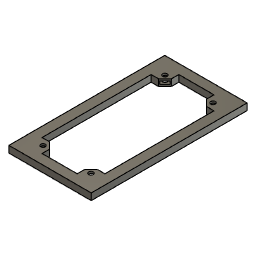
Dimensionen (Autodesk Fusion 360 design; units mm, degrees)
Autodesk Fusion 360 part; units mm, degrees
sketch "Einschubmuttern" plane through (0, 0, 0) normal (0, 1, 0) x (1, 0, 0)
  line L0 (2, 1.1547) -> (0, 2.3094)
  line L1 (0, 2.3094) -> (-2, 1.1547)
  line L2 (-2, 1.1547) -> (-2, -1.1547)
  line L3 (-2, -1.1547) -> (0, -2.3094)
  line L4 (0, -2.3094) -> (2, -1.1547)
  line L5 (2, -1.1547) -> (2, 1.1547)
  line L6 (9.3136, -1.6166) -> (12.1136, -3.2332)
  line L7 (12.1136, -3.2332) -> (14.9136, -1.6166)
  line L8 (14.9136, -1.6166) -> (14.9136, 1.6166)
  line L9 (14.9136, 1.6166) -> (12.1136, 3.2332)
  line L10 (12.1136, 3.2332) -> (9.3136, 1.6166)
  line L11 (9.3136, 1.6166) -> (9.3136, -1.6166)
  circle A0 centre (0, 0) radius 1.15
  circle A1 centre (12.1136, 0) radius 1.65
  circle A2 centre (0, 0) radius 2.25
  circle A3 centre (12.1136, 0) radius 3.25
  line L12 (3.3487, 2.8777) -> (-3.3487, 2.8777)
  line L13 (-3.3487, 2.8777) -> (-3.3487, -2.8777)
  line L14 (-3.3487, -2.8777) -> (3.3487, -2.8777)
  line L15 (3.3487, -2.8777) -> (3.3487, 2.8777)
  line L16 (16.2413, 3.8797) -> (7.986, 3.8797)
  line L17 (7.986, 3.8797) -> (7.986, -3.8797)
  line L18 (7.986, -3.8797) -> (16.2413, -3.8797)
  line L19 (16.2413, -3.8797) -> (16.2413, 3.8797)
  line L20 (-2, 1.1547) -> (-2, 2.8777)
  line L21 (2, 1.1547) -> (2, 2.8777)
  line L22 (9.3136, 1.6166) -> (9.3136, 3.8797)
  line L23 (14.9136, 1.6166) -> (14.9136, 3.8797)
  point P0 (12.1136, 0)
  point P1 (12.1136, 0)
  dimension "d1" = 2
  dimension "d2" = 2.8
  dimension "d3" = 2.3
  dimension "d4" = 3.3
  dimension "d5" = 4.5
  dimension "d6" = 6.5
  constraint coincident A0.centre A2.centre
  constraint coincident P1 P0
  constraint concentric A0 A2
  constraint concentric A1 A3
  constraint horizontal L12
  constraint perpendicular L12 L13
  constraint parallel L12 L14
  constraint parallel L13 L15
  constraint horizontal L16
  constraint perpendicular L16 L17
  constraint parallel L16 L18
  constraint parallel L17 L19
  constraint coincident L12 L20.end
  constraint perpendicular L12 L20
  constraint parallel L5 L21
  constraint coincident L16 L22.end
  constraint perpendicular L16 L22
  constraint coincident L16 L23.end
  constraint perpendicular L16 L23
  measures "d1" distance of A0.centre L5
  measures "d2" distance of P1 L11
  measures "d3" diameter of A0
  measures "d4" diameter of A1
  measures "d5" diameter of A2
  measures "d6" diameter of A3
extrude "Extrude1" add sketch "Einschubmuttern" against normal blind 5 contours L0 L5 A2 | L2 L3 L4 L5 A2 L12 L13 L14 L15 L20 L21 | L0 L1 A2 L12 L20 L21 | L0 L1 L2 L3 L4 L5 A2 | L0 A2 | L5 A2 | L0 L1 A2 | L4 L5 A2 | L1 A2 | L4 A2 | L1 L2 A2 | L3 L4 A2 | L2 A2 | L3 A2 | L2 L3 A2 makes body 1
extrude "Extrude2" cut sketch "Einschubmuttern" against normal blind 1.6 from surface at -2.5 contours L0 L5 A2 | L0 L1 A2 L12 L20 L21 | L0 L1 L2 L3 L4 L5 A2 | L0 A2 | L0 L1 A2 | L4 L5 A2 | L1 A2 | L1 L2 A2 | L3 L4 A2 | L2 L3 A2 bodies 1
extrude "Extrude3" add sketch "Einschubmuttern" against normal blind 6 separate body contours L6 L7 L8 L9 L10 L11 | L6 L7 L8 L11 A3 L22 L23 | L9 L10 A3 L22 L23 | A3 L16 L22 L23 | A3 L16 L17 L18 L19 L22 L23 makes body 2
extrude "Extrude4" cut sketch "Einschubmuttern" against normal blind 2.5 from surface at -3 contours L6 L7 L8 L9 L10 L11 | L9 L10 A3 L22 L23 | A3 L16 L22 L23 bodies 2
chamfer "Chamfer1" distance 1.1 angle 45 1 edges at (-1.0722, 0, -0.4159) on bodies 1
chamfer "Chamfer2" distance 1.6 angle 45 1 edges at (10.5753, 0, -0.5967) on bodies 2
sketch "Sketch2" plane through (0, 0, 0) normal (0, 1, 0) x (1, 0, 0)
  line L0 (2.25, 1.299) -> (0, 2.5981)
  line L1 (0, 2.5981) -> (-2.25, 1.299)
  line L2 (-2.25, 1.299) -> (-2.25, -1.299)
  line L3 (-2.25, -1.299) -> (0, -2.5981)
  line L4 (0, -2.5981) -> (2.25, -1.299)
  line L5 (2.25, -1.299) -> (2.25, 1.299)
  line L6 (14.5056, -1.5877) -> (17.2556, -3.1754)
  line L7 (17.2556, -3.1754) -> (20.0056, -1.5877)
  line L8 (20.0056, -1.5877) -> (20.0056, 1.5877)
  line L9 (20.0056, 1.5877) -> (17.2556, 3.1754)
  line L10 (17.2556, 3.1754) -> (14.5056, 1.5877)
  line L11 (14.5056, 1.5877) -> (14.5056, -1.5877)
  circle A0 centre (0, 0) radius 1.15
  circle A1 centre (17.2556, 0) radius 1.65
  line L12 (5.0227, 4.2637) -> (-5.0227, 4.2637)
  line L13 (-5.0227, 4.2637) -> (-5.0227, -4.2637)
  line L14 (-5.0227, -4.2637) -> (5.0227, -4.2637)
  line L15 (5.0227, -4.2637) -> (5.0227, 4.2637)
  line L16 (11.8758, 5.045) -> (22.6354, 5.045)
  line L17 (22.6354, 5.045) -> (22.6354, -5.045)
  line L18 (22.6354, -5.045) -> (11.8758, -5.045)
  line L19 (11.8758, -5.045) -> (11.8758, 5.045)
  point P0 (17.2556, 0)
  point P1 (17.2556, 0)
  dimension "d19" = 2.25
  dimension "d20" = 2.75
  dimension "d21" = 2.3
  dimension "d22" = 3.3
  constraint coincident A0.centre origin
  constraint coincident P1 P0
  constraint horizontal L12
  constraint perpendicular L12 L13
  constraint parallel L12 L14
  constraint parallel L13 L15
  constraint horizontal L16
  constraint perpendicular L16 L17
  constraint parallel L16 L18
  constraint parallel L17 L19
  measures "d19" distance of A0.centre L5
  measures "d20" distance of P1 L11
  measures "d21" diameter of A0
  measures "d22" diameter of A1
extrude "Extrude5" add sketch "Sketch2" against normal blind 3.5 separate body contours L0 L1 L2 L3 L4 L5 | L6 L7 L8 L9 L10 L11 | L12 L13 L14 L15 | L16 L17 L18 L19 makes body 3 at (3.7318, 0, 0) makes body 4 at (13.1191, 0, 0)
extrude "Extrude6" cut sketch "Sketch2" against normal blind 1.8 contours L0 L1 L2 L3 L4 L5 bodies 3
extrude "Extrude7" cut sketch "Sketch2" against normal blind 2.5 contours L6 L7 L8 L9 L10 L11 bodies 4
sketch "TOF" plane through (0, 0, 0) normal (0, 1, 0) x (1, 0, 0)
  line L0 (5.5969, 3.1885) -> (5.5969, 0.7636)
  line L1 (-8.8031, 0.7636) -> (-6.7031, -0.4488)
  line L2 (8.1469, -1.524) -> (8.1469, -1.6348)
  circle A0 centre (-1.8031, 1.976) radius 2.6
  line L3 (-6.7031, 4.4009) -> (-8.8031, 3.1885)
  line L4 (-9.6031, 2.476) -> (-9.6031, 1.476)
  line L5 (9.7969, 3.1885) -> (7.6969, 4.4009)
  circle A1 centre (7.6969, 1.976) radius 1.15
  arc A2 (-9.6031, 1.476) -> (-7.3062, -1.4404) centre (-6.6031, 1.476) ccw
  line L6 (-15.7687, -9.3798) -> (-15.7687, 8.4065)
  line L7 (0.4969, -1.524) -> (-7.1531, -1.524)
  line L8 (-8.8031, 3.1885) -> (-8.8031, 0.7636)
  line L9 (-7.1531, -1.524) -> (-7.1531, -1.6348)
  line L10 (5.5969, 0.7636) -> (7.6969, -0.4488)
  line L11 (5.3969, -0.624) -> (5.3969, 4.576)
  line L12 (-4.4031, 1.976) -> (-1.8031, 1.976)
  line L13 (0.4969, -6.024) -> (0.4969, -1.524)
  line L14 (-6.7031, -0.4488) -> (-4.6031, 0.7636)
  arc A3 (8.3, -1.4404) -> (8.1469, -1.6348) centre (8.3469, -1.6348) ccw
  circle A4 centre (-6.7031, 1.976) radius 1.15
  circle A5 centre (-6.7031, 1.976) radius 2.3
  line L15 (-4.4031, -0.624) -> (5.3969, -0.624)
  circle A6 centre (2.7969, 1.976) radius 2.6
  line L16 (-15.7687, 8.4065) -> (15.9174, 8.4065)
  line L17 (9.7969, 0.7636) -> (9.7969, 3.1885)
  line L18 (-4.4031, 4.576) -> (-4.4031, -0.624)
  arc A7 (-6.6031, 5.476) -> (-9.6031, 2.476) centre (-6.6031, 2.476) ccw
  arc A8 (10.5969, 2.476) -> (7.5969, 5.476) centre (7.5969, 2.476) ccw
  circle A9 centre (7.6969, 1.976) radius 2.3
  line L19 (-4.6031, 3.1885) -> (-6.7031, 4.4009)
  line L20 (-7.1531, -6.024) -> (0.4969, -6.024)
  line L21 (15.9174, 8.4065) -> (15.9174, -9.3798)
  line L22 (8.1469, -6.024) -> (0.4969, -6.024)
  line L23 (10.5969, 1.476) -> (10.5969, 2.476)
  line L24 (7.6969, -0.4488) -> (9.7969, 0.7636)
  line L25 (-7.1531, -1.524) -> (-7.1531, -6.024)
  line L26 (5.3969, 4.576) -> (-4.4031, 4.576)
  line L27 (5.3969, 1.976) -> (2.7969, 1.976)
  line L28 (-4.6031, 0.7636) -> (-4.6031, 3.1885)
  line L29 (8.1469, -1.524) -> (8.1469, -6.024)
  arc A10 (8.3, -1.4404) -> (10.5969, 1.476) centre (7.5969, 1.476) ccw
  line L30 (7.5969, 5.476) -> (-6.6031, 5.476)
  line L31 (7.6969, 4.4009) -> (5.5969, 3.1885)
  line L32 (-6.7031, 1.976) -> (7.6969, 1.976)
  arc A11 (-7.1531, -1.6348) -> (-7.3062, -1.4404) centre (-7.3531, -1.6348) ccw
  line L33 (15.9174, -9.3798) -> (-15.7687, -9.3798)
  line L34 (-6.6031, -1.524) -> (7.5969, -1.524)
  line L35 (0.4969, -6.024) -> (0.4969, -1.524)
  line L36 (0.4969, -1.524) -> (8.1469, -1.524)
  point P0 (0.4969, 1.976)
  point P1 (0.4969, 1.976)
  point P2 (7.6969, 1.976)
  point P3 (-6.7031, 1.976)
  dimension "d29" = 2.3
  dimension "d30" = 14.4
  dimension "d31" = 2.3
  dimension "d32" = 9.8
  dimension "d33" = 5.2
  dimension "d34" = 2.6
  dimension "d35" = 2.6
  dimension "d38" = 3
  dimension "d39" = 7.65
  dimension "d40" = 4.5
  dimension "d41" = 7.65
  dimension "d42" = 0.2
  dimension "d43" = 0.2
  dimension "d44" = 4.6
  dimension "d45" = 4.6
  dimension "d46" = 2.1
  dimension "d47" = 2.1
  constraint coincident P3 A4.centre
  constraint horizontal L32
  constraint coincident P2 A1.centre
  constraint horizontal L26
  constraint perpendicular L18 L26
  constraint parallel L15 L26
  constraint parallel L11 L18
  constraint midpoint P1 L32
  constraint midpoint L12.start L18
  constraint perpendicular L12 L18
  constraint coincident A0.centre L12.end
  constraint coincident L12.start A0
  constraint midpoint L27.start L11
  constraint perpendicular L11 L27
  constraint coincident A6.centre L27.end
  constraint coincident L27.start A6
  constraint horizontal L30
  constraint perpendicular L4 L30
  constraint parallel L30 L34
  constraint parallel L4 L23
  constraint coincident P1 P0
  constraint tangent A7 L30
  constraint tangent L4 A7
  constraint tangent A2 L34
  constraint tangent L4 A2
  constraint equal A2 A7
  constraint tangent A10 L34
  constraint tangent L23 A10
  constraint equal A7 A10
  constraint tangent A8 L30
  constraint tangent A8 L23
  constraint equal A7 A8
  constraint horizontal L36
  constraint vertical L29
  constraint horizontal L22
  constraint vertical L13
  constraint midpoint L7.start L34
  constraint horizontal L7
  constraint vertical L25
  constraint horizontal L20
  constraint vertical L35
  constraint perpendicular L7 L9
  constraint perpendicular L2 L36
  constraint tangent L2 A3
  constraint tangent A3 A10
  constraint tangent L9 A11
  constraint tangent A2 A11
  constraint horizontal L16
  constraint vertical L21
  constraint horizontal L33
  constraint vertical L6
  constraint coincident A1.centre A9.centre
  measures "d29" diameter of A4
  measures "d30" distance of P3 P2
  measures "d31" diameter of A1
  measures "d32" distance of L15.start L11.start
  measures "d33" distance of L15.start L18.start
  measures "d34" distance of L12.start A0.centre
  measures "d35" distance of A6.centre L27.start
  measures "d38" radius of A7
  measures "d39" distance of L7.start L2.start
  measures "d40" distance of L7.start L13.start
  measures "d41" distance of L7.start L7.end
  measures "d42" radius of A3
  measures "d43" radius of A11
  measures "d44" diameter of A5
  measures "d45" diameter of A9
  measures "d46" distance of P2 L17
  measures "d47" distance of P3 L28
extrude "TOF (1)" add sketch "TOF" against normal blind 1.3 separate body contours L0 A9 L31 | A5 L28 L32 | A5 L28 L32 | L11 L15 A6 | L11 A6 L26 | L0 L5 L10 L17 A9 L24 L31 | L0 A9 L32 | A9 L31 | L0 A9 L32 | L5 A9 L31 | L0 L10 A9 | L5 A9 | L10 A9 | A0 L18 L26 | A0 L15 L18 | L5 L17 A9 | L10 A9 L24 | L17 A9 | A9 L24 | L1 L3 L8 L14 A5 L19 L28 | A5 L19 L28 | L14 A5 L28 | L17 A9 L24 | A5 L19 | L14 A5 | L3 A5 L19 | L1 L14 A5 | L3 A5 | L1 A5 | L3 L8 A5 | L1 L8 A5 | L8 A5 | L2 L4 A2 L7 L9 A3 A7 A8 L23 L25 L29 A10 L30 A11 L34 L36 | L2 L13 L22 L29 L34 L35 L36 | L7 L9 L13 L20 L25 L34 L35 | L6 L16 L21 L33 makes body 5
extrude "TOF (2)" add sketch "TOF" along normal blind 2 contours L6 L16 L21 L33 bodies 5
chamfer "TOF (3)" distance 1.15 angle 45 2 edges at (-7.7753, -1.3, -1.5602) (6.6247, -1.3, -1.5602) on bodies 5
sketch "USB-C Buchse" plane through (0, 0, 0) normal (0, 1, 0) x (1, 0, 0)
  line L0 (0, 0) -> (14.25, 0)
  line L1 (14.25, 0) -> (14.25, -5.7)
  line L2 (14.25, -5.7) -> (0, -5.7)
  line L3 (0, -5.7) -> (0, 0)
  line L4 (20.5801, -12.0301) -> (-6.3301, -12.0301)
  line L5 (-6.3301, -12.0301) -> (-6.3301, 6.3301)
  line L6 (-6.3301, 6.3301) -> (20.5801, 6.3301)
  line L7 (20.5801, 6.3301) -> (20.5801, -12.0301)
  dimension "d53" = 14.25
  dimension "d54" = 5.7
  dimension "d55" = -6.3301
  constraint horizontal L0
  constraint vertical L1
  constraint horizontal L2
  constraint vertical L3
  constraint coincident L0.start L3.end
  measures "d53" distance of L0.start L0.end
  measures "d54" distance of L0.start L2.end
extrude "Extrude10" add sketch "USB-C Buchse" against normal blind 3 separate body makes body 6
sketch "USB-C Stecker" plane through (0, 0, 0) normal (0, 1, 0) x (1, 0, 0)
  line L0 (0, 0) -> (9, 0)
  line L1 (9, 0) -> (9, -3) construction
  line L2 (9, -3) -> (0, -3)
  line L3 (0, -3) -> (0, 0) construction
  line L4 (12, -6) -> (-3, -6)
  line L5 (-3, -6) -> (-3, 3)
  line L6 (-3, 3) -> (12, 3)
  line L7 (12, 3) -> (12, -6)
  line L8 (0, -1.5) -> (1.5, -1.5) construction
  line L9 (9, -1.5) -> (7.5, -1.5) construction
  circle A0 centre (1.5, -1.5) radius 1.5
  circle A1 centre (7.5, -1.5) radius 1.5
  dimension "d58" = 9
  dimension "d59" = 3
  dimension "d60" = -3
  dimension "d61" = 1.5
  dimension "d62" = 1.5
  constraint horizontal L0
  constraint vertical L1
  constraint horizontal L2
  constraint vertical L3
  constraint coincident L0.start L3.end
  constraint midpoint L3 L8.start
  constraint perpendicular L3 L8
  constraint midpoint L1 L9.start
  constraint perpendicular L1 L9
  constraint coincident L8.end A0.centre
  constraint coincident L8.start A0
  constraint coincident L9.end A1.centre
  constraint coincident L9.start A1
  measures "d58" distance of L0.start L0.end
  measures "d59" distance of L0.start L2.end
  measures "d61" distance of L8.start L8.end
  measures "d62" distance of L9.start L9.end
extrude "Extrude11" add sketch "USB-C Stecker" against normal blind 3 separate body makes body 7
sketch "ESP32-C6-DevKit" plane through (0, 0, 0) normal (0, 1, 0) x (1, 0, 0)
  circle A0 centre (24.0333, -6.3894) radius 1.25
  circle A1 centre (24.0333, -27.2477) radius 1.25
  line L0 (28.261, -31.6633) -> (-30.2467, -31.6633)
  line L1 (-29.9467, -3.9685) -> (-29.9467, -29.6686)
  line L2 (28.261, -3.3133) -> (28.261, -31.6633)
  line L3 (30.5691, -27.2494) -> (24.0333, -27.2494) construction
  circle A2 centre (-27.1863, -27.2477) radius 1.25
  line L4 (26.761, -3.9685) -> (-29.9467, -3.9685)
  line L5 (26.761, -29.6686) -> (26.761, -3.9685)
  line L6 (-28.9563, -27.2477) -> (25.1533, -27.2477) construction
  line L7 (28.261, -2.4685) -> (-30.5467, -2.4685)
  line L8 (25.1533, -6.3894) -> (-28.9563, -6.3894) construction
  line L9 (-29.9467, -29.6686) -> (26.761, -29.6686)
  circle A3 centre (-27.1863, -6.3894) radius 1.25
  line L10 (-29.3467, -29.6686) -> (-29.9467, -29.6686)
  line L11 (24.0333, -5.1352) -> (24.0333, -29.4977) construction
  line L12 (-29.6467, -3.9685) -> (-29.9467, -3.9685)
  line L13 (25.1533, -14.9026) -> (25.1533, -6.3894) construction
  line L14 (-27.1863, -5.1352) -> (-27.1863, -29.4977) construction
  line L15 (-28.9563, -6.3894) -> (-28.9563, -27.2477) construction
  line L16 (30.5691, -6.3894) -> (30.5691, -27.2494) construction
  line L17 (24.0333, -27.2494) -> (24.0333, -6.3894) construction
  line L18 (24.0333, -6.3894) -> (30.5691, -6.3894) construction
  line L19 (-27.1863, -25.0177) -> (-27.0488, -25.0177)
  line L20 (28.261, -3.3133) -> (28.261, -2.4685)
  line L21 (-25.1863, -5.2347) -> (-27.1863, -4.08)
  line L22 (-27.1863, -4.08) -> (-29.1863, -5.2347)
  line L23 (-29.1863, -5.2347) -> (-29.1863, -7.5441)
  line L24 (-29.1863, -7.5441) -> (-27.1863, -8.6988)
  line L25 (-27.1863, -8.6988) -> (-25.1863, -7.5441)
  line L26 (-25.1863, -7.5441) -> (-25.1863, -5.2347)
  line L27 (-25.1863, -5.2347) -> (-25.1863, -2.4685)
  line L28 (-29.1863, -5.2347) -> (-29.1863, -2.4685)
  line L29 (26.0333, -5.2347) -> (24.0333, -4.08)
  line L30 (24.0333, -4.08) -> (22.0333, -5.2347)
  line L31 (22.0333, -5.2347) -> (22.0333, -7.5441)
  line L32 (22.0333, -7.5441) -> (24.0333, -8.6988)
  line L33 (24.0333, -8.6988) -> (26.0333, -7.5441)
  line L34 (26.0333, -7.5441) -> (26.0333, -5.2347)
  line L35 (26.0344, -26.0949) -> (24.0354, -24.9383)
  line L36 (24.0354, -24.9383) -> (22.0344, -26.0912)
  line L37 (22.0344, -26.0912) -> (22.0322, -28.4006)
  line L38 (22.0322, -28.4006) -> (24.0312, -29.5571)
  line L39 (24.0312, -29.5571) -> (26.0322, -28.4043)
  line L40 (26.0322, -28.4043) -> (26.0344, -26.0949)
  line L41 (-25.1863, -26.093) -> (-27.1863, -24.9383)
  line L42 (-27.1863, -24.9383) -> (-29.1863, -26.093)
  line L43 (-29.1863, -26.093) -> (-29.1863, -28.4024)
  line L44 (-29.1863, -28.4024) -> (-27.1863, -29.5571)
  line L45 (-27.1863, -29.5571) -> (-25.1863, -28.4024)
  line L46 (-25.1863, -28.4024) -> (-25.1863, -26.093)
  line L47 (-25.1863, -28.4024) -> (-25.1863, -31.6633)
  line L48 (-29.1863, -28.4024) -> (-29.1863, -31.6633)
  line L49 (22.0333, -5.2347) -> (22.0333, -2.4685)
  line L50 (26.0333, -5.2347) -> (26.0333, -2.4685)
  line L51 (26.0322, -28.4043) -> (26.0322, -31.6633)
  line L52 (22.0322, -28.4006) -> (22.0322, -31.6633)
  line L53 (-29.9467, -17.4783) -> (-30.5467, -17.4783)
  line L54 (-30.5467, -21.9783) -> (-29.9467, -21.9783)
  line L55 (-29.9467, -21.9783) -> (-29.9467, -17.4783)
  line L56 (-29.9467, -17.4783) -> (-30.5467, -17.4783)
  line L57 (-30.5467, -12.9783) -> (-29.9467, -12.9783)
  line L58 (-29.9467, -12.9783) -> (-29.9467, -17.4783)
  line L59 (-24.9563, -29.6686) -> (-24.7063, -29.6686)
  line L60 (-24.7063, -29.6686) -> (-24.7063, -4.4633)
  line L61 (21.6533, -3.9685) -> (21.4033, -3.9685)
  line L62 (-24.7063, -4.4633) -> (-24.7063, -3.9685)
  line L63 (21.5526, -3.9685) -> (21.5526, -29.6686)
  line L64 (-30.5467, -2.4685) -> (-30.7467, -2.4685)
  line L65 (-30.7467, -2.4685) -> (-30.7467, -31.6633)
  line L66 (-30.7467, -31.6633) -> (-30.2467, -31.6633)
  line L67 (-30.5467, -12.9783) -> (-30.7467, -12.9783)
  line L68 (-30.5467, -21.9783) -> (-30.7467, -21.9783)
  line L69 (-30.5467, -17.4783) -> (-30.7467, -17.4783)
  point P0 (-28.9563, -17.3164)
  point P1 (-1.5967, -17.8133)
  point P2 (-28.9563, -29.4977)
  point P3 (-27.1863, -6.3894)
  point P4 (24.0333, -6.3894)
  point P5 (24.0333, -27.2477)
  point P6 (-27.1863, -27.2477)
  dimension "d67" = 2.5
  dimension "d68" = 2.5
  dimension "d69" = 2.5
  dimension "d70" = 2.5
  dimension "d137" = 20.86
  dimension "d138" = 2
  dimension "d139" = 2
  dimension "d140" = 2
  dimension "d141" = 2
  dimension "d142" = 4.5
  dimension "d143" = 4.5
  constraint horizontal L8
  constraint perpendicular L8 L15
  constraint parallel L13 L15
  constraint horizontal L6
  constraint vertical L11
  constraint vertical L14
  constraint coincident P3 L14
  constraint coincident P3 L8
  constraint coincident P4 L8
  constraint coincident P4 L11
  constraint coincident P5 L6
  constraint coincident P5 L11
  constraint coincident P6 L6
  constraint coincident P6 L14
  constraint horizontal L4
  constraint parallel L4 L9
  constraint horizontal L12
  constraint vertical L1
  constraint horizontal L10
  constraint coincident L12.start L4
  constraint coincident L10.start L9
  constraint horizontal L0
  constraint vertical L2
  constraint coincident L59.start L9
  constraint coincident L19.start L14
  constraint coincident L61.start L4
  constraint horizontal L18
  constraint vertical L16
  constraint horizontal L3
  constraint vertical L17
  constraint coincident P4 A0.centre
  constraint perpendicular L7 L20
  constraint coincident P3 A3.centre
  constraint coincident L7 L27.end
  constraint perpendicular L7 L27
  constraint coincident L7 L28.end
  constraint perpendicular L7 L28
  constraint coincident P5 A1.centre
  constraint coincident P6 A2.centre
  constraint coincident L0 L47.end
  constraint perpendicular L0 L47
  constraint coincident L0 L48.end
  constraint perpendicular L0 L48
  constraint coincident L7 L49.end
  constraint perpendicular L7 L49
  constraint coincident L7 L50.end
  constraint perpendicular L7 L50
  constraint coincident L0 L51.end
  constraint perpendicular L0 L51
  constraint coincident L0 L52.end
  constraint perpendicular L0 L52
  constraint horizontal L53
  constraint horizontal L54
  constraint vertical L55
  constraint horizontal L56
  constraint horizontal L57
  constraint vertical L58
  constraint horizontal L59
  constraint vertical L60
  constraint horizontal L61
  constraint coincident L41 L19.end
  constraint coincident L4 L62.end
  constraint perpendicular L4 L62
  constraint coincident L4 L63.start
  constraint coincident L9 L63.end
  constraint perpendicular L9 L63
  constraint coincident L1 L53.start
  constraint horizontal L64
  constraint vertical L65
  constraint horizontal L66
  constraint coincident L65 L67.end
  constraint perpendicular L65 L67
  constraint coincident L65 L68.end
  constraint perpendicular L65 L68
  constraint coincident L65 L69.end
  constraint perpendicular L65 L69
  measures "d67" diameter of A3
  measures "d68" diameter of A0
  measures "d69" diameter of A1
  measures "d70" diameter of A2
  measures "d137" distance of L16.start L3.start
  measures "d138" distance of P3 L26
  measures "d139" distance of P4 L34
  measures "d140" distance of P5 L40
  measures "d141" distance of P6 L46
  measures "d142" distance of L53.start L54.end
  measures "d143" distance of L53.start L57.end
extrude "Boden" add sketch "ESP32-C6-DevKit" against normal blind 1 separate body makes body 8
extrude "Ablage" add sketch "ESP32-C6-DevKit" along normal blind 9.3 contours L4 L5 L9 L31 L32 L33 L34 L35 L36 L37 L40 L49 L50 L51 L52 L61 L63 | L9 L38 L39 L51 L52 | L35 L36 L37 L38 L39 L40 | L1 L4 L9 L10 L12 L23 L24 L25 L26 L27 L28 L41 L42 L43 L46 L47 L48 L55 L58 L59 L60 L62 | L9 L44 L45 L47 L48 | L4 L29 L30 L49 L50 | L41 L42 L43 L44 L45 L46 | L29 L30 L31 L32 L33 L34 | L4 L21 L22 L27 L28 | L21 L22 L23 L24 L25 L26 bodies 8
extrude "Extrude15" add sketch "ESP32-C6-DevKit" along normal blind 15.9 contours L0 L2 L4 L5 L7 L9 L20 L50 L51 | L0 L9 L51 L52 | L0 L9 L47 L52 L59 | L0 L9 L47 L48 | L4 L7 L49 L50 | L0 L1 L9 L10 L48 L54 L65 L66 L68 | L4 L7 L27 L49 L61 | L4 L7 L27 L28 | L1 L4 L7 L12 L28 L57 L64 L65 L67 | L1 L53 L54 L55 L56 L65 L68 L69 | L1 L53 L56 L57 L58 L65 L67 L69 bodies 8
extrude "Einschubmutter" cut sketch "ESP32-C6-DevKit" against normal blind 1.6 from surface at 8.3 contours L0 L9 L51 L52 | L9 L38 L39 L51 L52 | L0 L9 L47 L48 | L35 L36 L37 L38 L39 L40 | L4 L7 L49 L50 | L9 L44 L45 L47 L48 | L4 L29 L30 L49 L50 | L41 L42 L43 L44 L45 L46 | L4 L7 L27 L28 | L29 L30 L31 L32 L33 L34 | L4 L21 L22 L27 L28 | L21 L22 L23 L24 L25 L26 bodies 8
sketch "ESP32-DevKit Wand Buchse" plane through (-30.7467, 0, 0) normal (-1, 0, 0) x (0, 0, 1)
  line L0 (2.4685, 15.9) -> (2.4685, -1)
  line L1 (2.4685, -1) -> (31.6633, -1)
  line L2 (31.6633, -1) -> (31.6633, 15.9)
  line L3 (31.6633, 15.9) -> (2.4685, 15.9)
  line L4 (3.9685, 9.3) -> (29.6686, 9.3)
  line L5 (12.3186, 9.3) -> (21.078, 9.3)
  line L6 (21.078, 10.9) -> (12.3186, 10.9)
  line L7 (12.3186, 10.9) -> (12.3186, 9.3)
  line L8 (12.3186, 10.9) -> (21.3186, 10.9)
  line L9 (21.3186, 10.9) -> (21.3186, 13.9)
  line L10 (21.3186, 13.9) -> (12.3186, 13.9)
  line L11 (12.3186, 13.9) -> (12.3186, 10.9)
  line L12 (12.3186, 12.4) -> (13.8186, 12.4)
  circle A0 centre (13.8186, 12.4) radius 1.5
  line L13 (21.3186, 12.4) -> (19.8186, 12.4)
  circle A1 centre (19.8186, 12.4) radius 1.5
  dimension "d271" = 1.6
  dimension "d272" = 3
  dimension "d273" = 1.5
  dimension "d274" = 1.5
  constraint horizontal L5
  constraint horizontal L6
  constraint vertical L7
  constraint coincident L4 L5.start
  constraint horizontal L8
  constraint vertical L9
  constraint horizontal L10
  constraint vertical L11
  constraint midpoint L11 L12.start
  constraint perpendicular L11 L12
  constraint coincident L12.end A0.centre
  constraint coincident L12.start A0
  constraint midpoint L9 L13.start
  constraint perpendicular L9 L13
  constraint coincident L13.end A1.centre
  constraint coincident L13.start A1
  measures "d271" distance of L5.start L6.end
  measures "d272" distance of L6.end L10.end
  measures "d273" distance of L12.start L12.end
  measures "d274" distance of L13.start L13.end
extrude "Extrude27" cut sketch "ESP32-DevKit Wand Buchse" along normal mid plane 6 contours L6 L8 L10 A0 A1 | A1 | A0 bodies 8
sketch "LED-Ring" plane through (0, 0, 0) normal (0, 1, 0) x (1, 0, 0)
  circle A0 centre (0, 0) radius 18
  circle A1 centre (0, 0) radius 20.7 construction
  line L0 (0, 0) -> (0, -20.7) construction
  line L1 (2.8, -17.9) -> (-2.8, -17.9)
  line L2 (-2.8, -17.9) -> (-2.8, -23.5)
  line L3 (-2.8, -23.5) -> (2.8, -23.5)
  line L4 (2.8, -23.5) -> (2.8, -17.9)
  line L5 (2.8, -17.9) -> (-2.8, -23.5) construction
  line L6 (-2.8, -17.9) -> (2.8, -23.5) construction
  circle A2 centre (0, -20.7) radius 1.75
  line L7 (0, 0) -> (22.6032, -22.6032) construction
  line L8 (0, 0) -> (31.9658, 0) construction
  circle A3 centre (0, 0) radius 23.18 construction
  circle A4 centre (16.3907, -16.3907) radius 1.25
  circle A5 centre (0, 0) radius 32.5
  circle A6 centre (16.3907, -16.3907) radius 2.25
  line L9 (7.6403, -23.8039) -> (7.6403, -31.5892)
  line L10 (-7.6403, -31.5892) -> (-7.6403, -23.8039)
  arc A7 (-7.6403, -23.8039) -> (7.6403, -23.8039) centre (0, 0) ccw
  arc A8 (17.6777, -17.6777) -> (16.6799, -18.6221) centre (0, 0) ccw
  line L11 (-2.8, -23.5) -> (2.8, -23.5)
  line L12 (2.8, -23.5) -> (2.8, -25.3)
  line L13 (2.8, -25.3) -> (-2.8, -25.3)
  line L14 (-2.8, -25.3) -> (-2.8, -23.5)
  point P0 (0, -20.7)
  point P1 (0, -25)
  dimension "d170" = 50
  dimension "d171" = 36
  dimension "d172" = 2.7
  dimension "d173" = 5.6
  dimension "d174" = 5.6
  dimension "d175" = 3.5
  dimension "d176" = 45
  dimension "d178" = 2.5
  dimension "d179" = 65
  dimension "d190" = 4.5
  dimension "d267" = 1.8
  constraint coincident A0.centre A1.centre
  constraint concentric A0 A8
  constraint coincident A1 P0
  constraint vertical L0
  constraint horizontal L1
  constraint perpendicular L1 L2
  constraint parallel L1 L3
  constraint parallel L2 L4
  constraint coincident L5 P0
  constraint coincident L6 P0
  constraint coincident P0 L0.end
  constraint horizontal L8
  constraint coincident L7 A4.centre
  constraint coincident A3 A4.centre
  constraint concentric A5 A8
  constraint concentric A4 A6
  constraint parallel L9 L10
  constraint coincident P1 A8
  constraint coincident L9.start A8
  constraint coincident L10.end A8
  constraint coincident A5 L10.start
  constraint coincident A5 L9.end
  constraint coincident A6 A8.end
  constraint concentric A3 A8
  constraint coincident L7 A8.start
  constraint horizontal L11
  constraint vertical L12
  constraint horizontal L13
  constraint vertical L14
  measures "d170" diameter of A8
  measures "d171" diameter of A0
  measures "d173" distance of L2.end L3.end
  measures "d174" distance of L1.end L2.end
  measures "d175" diameter of A2
  measures "d176" angle of L7 L8
  measures "d178" diameter of A4
  measures "d179" diameter of A5
  measures "d190" diameter of A6
  measures "d267" distance of L2.end L13.end
extrude "LED-Ring Base Plate" add sketch "LED-Ring" against normal blind 2 separate body contours A0 L1 | A0 L1 L2 L4 A6 A7 A8 L12 L14 | A0 L1 | A0 L1 L2 L3 L4 L11 | L3 A7 A8 L11 L12 L14 | A5 L9 L10 A7 A8 L12 L13 L14 | A7 A8 L12 L13 L14 | A5 A6 L9 L10 A8 | A6 | A2 | A4 makes body 9
extrude "Lichtloch" cut sketch "LED-Ring" against normal blind 2 contours A2 bodies 9
pattern_circular "Löcher Lattern" count 12 over 360 about axis through (0, 0, 0) along (0, 1, 0) of "Lichtloch"
extrude "SMD Loch" cut sketch "LED-Ring" against normal blind 1.5 contours A0 L1 | A0 L1 L2 L3 L4 L11 | L3 A7 A8 L11 L12 L14 | A7 A8 L12 L13 L14 picked at (-0.2109, -17.9296) bodies 9
fillet "Fillet4" radius 1.6 2 edges at (2.8, -0.75, 25.3) (-2.8, -0.75, 25.3) on bodies 9
pattern_circular "SMD Aussparungen" count 12 over 360 about axis through (0, 0, 0) along (0, 1, 0) of "SMD Loch", "Fillet4"
extrude "Schraubenloch" cut sketch "LED-Ring" against normal blind 5 contours A4 bodies 9
chamfer "Chamfer4" distance 1 angle 45 1 edges at (15.2253, -2, 16.8428) on bodies 9
pattern_circular "C-Pattern3" count 4 over 360 about axis through (0, 0, 0) along (0, 1, 0) of "Schraubenloch", "Chamfer4"
extrude "Extrude21" cut sketch "LED-Ring" against normal blind 1.4 contours A5 L9 L10 A7 A8 L12 L13 L14 | A7 A8 L12 L13 L14 bodies 9
sketch "OLED SSD1306" plane through (0, 0, 0) normal (0, 1, 0) x (1, 0, 0)
  circle A0 centre (0, 0) radius 1.15
  line L0 (0, 0) -> (22, 0) construction
  line L1 (22, 0) -> (22, -22) construction
  line L2 (22, -22) -> (0, -22) construction
  line L3 (0, -22) -> (0, 0) construction
  circle A1 centre (22, 0) radius 1.15
  circle A2 centre (22, -22) radius 1.15
  circle A3 centre (0, -22) radius 1.15
  line L4 (-2.6, -24.6) -> (-2.6, 2.6)
  line L5 (-2.6, 2.6) -> (24.6, 2.6)
  line L6 (24.6, 2.6) -> (24.6, -24.6)
  line L7 (24.6, -24.6) -> (-2.6, -24.6)
  line L8 (-2.6, 2.6) -> (24.6, 2.6)
  line L9 (-2.6, -16.4) -> (-2.6, 2.6)
  line L10 (24.6, -2.7) -> (-2.6, -2.7)
  line L11 (-2.6, -2.7) -> (-2.6, -16.4)
  line L12 (29.4101, -27.9616) -> (-8.052, -27.9616)
  line L13 (-8.052, -27.9616) -> (-8.052, 5.9616)
  line L14 (-8.052, 5.9616) -> (29.4101, 5.9616)
  line L15 (29.4101, 5.9616) -> (29.4101, -27.9616)
  line L16 (29.4101, -27.9616) -> (-8.052, 5.9616) construction
  line L17 (-8.052, -27.9616) -> (29.4101, 5.9616) construction
  circle A4 centre (22, -22) radius 2.25 construction
  circle A5 centre (22, 0) radius 2.25 construction
  circle A6 centre (0, 0) radius 2.25 construction
  circle A7 centre (0, -22) radius 2.25 construction
  line L18 (-2.6, 2.6) -> (2, 2.6)
  line L19 (2, 2.6) -> (2, -2.7)
  line L20 (2, -2.7) -> (-2.6, -2.7)
  line L21 (-2.6, -2.7) -> (-2.6, 2.6)
  line L22 (24.6, 2.6) -> (20, 2.6)
  line L23 (20, 2.6) -> (20, -2.7)
  line L24 (20, -2.7) -> (24.6, -2.7)
  line L25 (24.6, -2.7) -> (24.6, 2.6)
  line L26 (24.6, -24.6) -> (20, -24.6)
  line L27 (24.6, -16.4) -> (24.6, -24.6)
  line L28 (2, -24.6164) -> (-2.6, -24.6164)
  line L29 (-2.6, -24.6164) -> (-2.6, -16.4)
  line L30 (24.6, -24.6) -> (-2.6, -24.6)
  line L31 (-2.6, -24.6) -> (-2.6, -19.3)
  line L32 (-2.6, -19.3) -> (24.6, -19.3)
  line L33 (24.6, -19.3) -> (24.6, -24.6)
  line L34 (2, -19.3) -> (2, -24.6164)
  line L35 (20, -24.6) -> (20, -19.3)
  line L36 (24.6, -2.7) -> (19.6, -2.7)
  line L37 (19.6, -2.7) -> (19.6, -2)
  line L38 (19.6, -2) -> (24.6, -2)
  line L39 (24.6, -2) -> (24.6, -2.7)
  line L40 (2, -2.7) -> (-2.6, -2.7)
  line L41 (-2.6, -2.7) -> (-2.6, -2)
  line L42 (-2.6, -2) -> (2, -2)
  line L43 (2, -2) -> (2, -2.7)
  line L44 (2, -19.3) -> (-2.6, -19.3)
  line L45 (-2.6, -19.3) -> (-2.6, -20)
  line L46 (-2.6, -20) -> (2, -20)
  line L47 (2, -20) -> (2, -19.3)
  line L48 (24.6, -19.3) -> (19.6, -19.3)
  line L49 (19.6, -19.3) -> (19.6, -20)
  line L50 (19.6, -20) -> (24.6, -20)
  line L51 (24.6, -20) -> (24.6, -19.3)
  point P0 (10.679, -11)
  dimension "d198" = 2.3
  dimension "d199" = 22
  dimension "d200" = 22
  dimension "d201" = 2.3
  dimension "d202" = 2.3
  dimension "d203" = 2.3
  dimension "d204" = -2.6
  dimension "d209" = 4.5
  dimension "d210" = 4.5
  dimension "d211" = 4.5
  dimension "d212" = 4.5
  dimension "d216" = 4.6
  dimension "d217" = 4.6
  dimension "d218" = 4.6
  dimension "d255" = 5.3
  dimension "d256" = 4.6
  dimension "d257" = 0.7
  dimension "d258" = 0.7
  dimension "d259" = 0.7
  dimension "d260" = 0.7
  dimension "d263" = 4.6
  constraint coincident A0.centre L0.start
  constraint horizontal L0
  constraint vertical L1
  constraint horizontal L2
  constraint vertical L3
  constraint coincident L0.end L1.start
  constraint coincident L1.end L2.start
  constraint coincident L2.end L3.start
  constraint horizontal L8
  constraint vertical L9
  constraint horizontal L10
  constraint vertical L11
  constraint coincident L6 L10.start
  constraint horizontal L12
  constraint perpendicular L12 L13
  constraint parallel L12 L14
  constraint parallel L13 L15
  constraint coincident L16 P0
  constraint coincident L17 P0
  constraint concentric A2 A4
  constraint concentric A1 A5
  constraint concentric A3 A7
  constraint horizontal L18
  constraint vertical L19
  constraint horizontal L20
  constraint vertical L21
  constraint horizontal L22
  constraint vertical L23
  constraint horizontal L24
  constraint vertical L25
  constraint horizontal L26
  constraint vertical L35
  constraint vertical L27
  constraint horizontal L28
  constraint vertical L29
  constraint horizontal L30
  constraint vertical L31
  constraint horizontal L32
  constraint vertical L33
  constraint coincident L32 L34.start
  constraint coincident L32 L35.end
  constraint horizontal L36
  constraint vertical L37
  constraint horizontal L38
  constraint vertical L39
  constraint horizontal L40
  constraint vertical L41
  constraint horizontal L42
  constraint vertical L43
  constraint horizontal L44
  constraint vertical L45
  constraint horizontal L46
  constraint vertical L47
  constraint horizontal L48
  constraint vertical L49
  constraint horizontal L50
  constraint vertical L51
  measures "d198" diameter of A0
  measures "d199" distance of A0.centre L0.end
  measures "d200" distance of A0.centre L2.end
  measures "d201" diameter of A1
  measures "d202" diameter of A2
  measures "d203" diameter of A3
  measures "d209" diameter of A4
  measures "d210" diameter of A5
  measures "d211" diameter of A6
  measures "d212" diameter of A7
  measures "d216" distance of L4.end L18.end
  measures "d217" distance of L5.end L22.end
  measures "d218" distance of L6.end L26.end
  measures "d255" distance of L6.end L32.end
  measures "d256" distance of L28.start L28.end
  measures "d257" distance of L10.start L38.end
  measures "d258" distance of L19.end L42.end
  measures "d259" distance of L34.start L46.end
  measures "d260" distance of L32.end L50.end
  measures "d263" distance of L45.end L46.end
extrude "Grundplatte" add sketch "OLED SSD1306" against normal blind 3 separate body contours L4 L7 L29 L30 L31 L34 L46 | L7 L28 L29 L30 L34 | L4 L29 L31 L32 L34 L44 L45 L46 L47 | L7 L30 L32 L34 L35 L47 L49 L50 | L6 L7 L26 L27 L30 L33 L35 L50 | L32 L35 L48 L49 L50 | L6 L27 L32 L33 L35 L48 L50 L51 | L4 L9 L10 L19 L20 L21 L40 L41 L42 L43 | L4 L5 L8 L9 L18 L19 L21 L42 | L5 L8 L10 L19 L23 L37 L38 L43 | L10 L23 L36 L37 L38 | L6 L10 L23 L24 L25 L36 L38 L39 | L5 L6 L8 L22 L23 L25 L38 | L12 L13 L14 L15 makes body 10
extrude "Schrubsockel" cut sketch "OLED SSD1306" against normal blind 1.3 contours L4 L7 L29 L30 L31 L34 L46 | L4 L29 L31 L32 L34 L44 L45 L46 L47 | L7 L30 L32 L34 L35 L47 L49 L50 | L6 L7 L26 L27 L30 L33 L35 L50 | L32 L35 L48 L49 L50 | L6 L27 L32 L33 L35 L48 L50 L51 | L4 L9 L10 L19 L20 L21 L40 L41 L42 L43 | L4 L5 L8 L9 L18 L19 L21 L42 | L5 L8 L10 L19 L23 L37 L38 L43 | L10 L23 L36 L37 L38 | L6 L10 L23 L24 L25 L36 L38 L39 | L5 L6 L8 L22 L23 L25 L38 bodies 10
chamfer "Schraubenkopf" distance 1.1 angle 45 4 edges at (20.9278, -3, 22.4159) (-1.0722, -3, 22.4159) (-1.0722, -3, 0.4159) (20.9278, -3, 0.4159) on bodies 10
extrude "Platz für Anschlüsse" cut sketch "OLED SSD1306" against normal blind 2.4 contours L4 L29 L31 L32 L34 L44 L45 L46 L47 | L7 L30 L32 L34 L35 L47 L49 L50 | L32 L35 L48 L49 L50 | L6 L27 L32 L33 L35 L48 L50 L51 | L4 L9 L10 L19 L20 L21 L40 L41 L42 L43 | L5 L8 L10 L19 L23 L37 L38 L43 | L10 L23 L36 L37 L38 | L6 L10 L23 L24 L25 L36 L38 L39 bodies 10
extrude "enger links" add 1 faces at (14, -0.4333, 24.6) along direction (0, 0, -1) blind 0.3 on bodies 10 bodies 10
extrude "enger rechts" add 1 faces at (8, -0.4333, -2.6) along direction (0, 0, 1) blind 0.3 on bodies 10 bodies 10
fillet "Fillet2" radius 2.75 4 edges at (20, -1.85, 20) (2, -1.85, 20) (2, -1.85, 2) (20, -1.85, 2) on bodies 10
fillet "Fillet3" radius 0.75 12 edges at (20, -2.4, -1.525) (20.8055, -2.4, 1.1945) (23.675, -2.4, 2) (23.675, -2.4, 20) (20.8055, -2.4, 20.8055) (20, -2.4, 23.525) (2, -2.4, 23.525) (1.1945, -2.4, 20.8055) (-1.675, -2.4, 20) (-1.675, -2.4, 2) (1.1945, -2.4, 1.1945) (2, -2.4, -1.525) on bodies 10
sketch "Platine 3*7" plane through (0, 0, 0) normal (0, 1, 0) x (1, 0, 0)
  circle A0 centre (0, 0) radius 1.25
  line L0 (0, 0) -> (-26, 0)
  line L1 (-26, 0) -> (-26, 66)
  line L2 (-26, 66) -> (0, 66)
  line L3 (0, 66) -> (0, 0)
  circle A1 centre (-26, 0) radius 1.25
  circle A2 centre (-26, 66) radius 1.25
  circle A3 centre (0, 66) radius 1.25
  circle A4 centre (0, 0) radius 3.5
  circle A5 centre (-26, 0) radius 3.5
  circle A6 centre (-26, 66) radius 3.5
  circle A7 centre (0, 66) radius 3.5
  line L4 (-28, -2) -> (2, -2) construction
  line L5 (2, -2) -> (2, 68) construction
  line L6 (2, 68) -> (-28, 68) construction
  line L7 (-28, 68) -> (-28, -2) construction
  line L8 (-28, -2) -> (2, 68) construction
  line L9 (2, -2) -> (-28, 68) construction
  line L10 (-30, 70) -> (-30, -4)
  line L11 (-30, -4) -> (4, -4)
  line L12 (4, -4) -> (4, 70)
  line L13 (4, 70) -> (-30, 70)
  line L14 (-35.2918, 75.1805) -> (9.2918, 75.1805)
  line L15 (9.2918, 75.1805) -> (9.2918, -9.1805)
  line L16 (9.2918, -9.1805) -> (-35.2918, -9.1805)
  line L17 (-35.2918, -9.1805) -> (-35.2918, 75.1805)
  line L18 (-26, 3.5) -> (-30, 3.5)
  line L19 (-22.5, 0) -> (-22.5, -4)
  line L20 (-3.5, 0) -> (-3.5, -4)
  line L21 (0, 3.5) -> (4, 3.5)
  line L22 (-26, 62.5) -> (-30, 62.5)
  line L23 (-22.5, 66) -> (-22.5, 70)
  line L24 (-3.5, 66) -> (-3.5, 70)
  line L25 (0, 62.5) -> (4, 62.5)
  line L26 (-26, 0) -> (-23.5251, -2.4749) construction
  line L27 (-26, 0) -> (-22.5, 0) construction
  line L28 (-23.7693, -0.5977) -> (-24.367, 1.633)
  line L29 (-24.367, 1.633) -> (-26.5977, 2.2307)
  line L30 (-26.5977, 2.2307) -> (-28.2307, 0.5977)
  line L31 (-28.2307, 0.5977) -> (-27.633, -1.633)
  line L32 (-27.633, -1.633) -> (-25.4023, -2.2307)
  line L33 (-25.4023, -2.2307) -> (-23.7693, -0.5977)
  line L34 (-23.7693, -0.5977) -> (-22.5548, 0.6168)
  line L35 (-26.5977, 2.2307) -> (-25.3832, 3.4452)
  line L36 (-26.5977, 2.2307) -> (-25.706, 2.2307) construction
  line L37 (0, 0) -> (2.4749, 2.4749) construction
  line L38 (0, 0) -> (3.5, 0) construction
  line L39 (0.5977, 2.2307) -> (-1.633, 1.633)
  line L40 (-1.633, 1.633) -> (-2.2307, -0.5977)
  line L41 (-2.2307, -0.5977) -> (-0.5977, -2.2307)
  line L42 (-0.5977, -2.2307) -> (1.633, -1.633)
  line L43 (1.633, -1.633) -> (2.2307, 0.5977)
  line L44 (2.2307, 0.5977) -> (0.5977, 2.2307)
  line L45 (-3.4452, 0.6168) -> (-2.2307, -0.5977)
  line L46 (2.2307, 0.5977) -> (-0.6168, 3.4452)
  line L47 (0, 3.5) -> (-3.5, 0)
  line L48 (-22.5, 0) -> (-26, 3.5)
  line L49 (-22.5, 66) -> (-26, 62.5)
  line L50 (-26, 66) -> (-23.5251, 68.4749) construction
  line L51 (-26, 66) -> (-22.5, 66) construction
  line L52 (-25.4023, 68.2307) -> (-27.633, 67.633)
  line L53 (-27.633, 67.633) -> (-28.2307, 65.4023)
  line L54 (-28.2307, 65.4023) -> (-26.5977, 63.7693)
  line L55 (-26.5977, 63.7693) -> (-24.367, 64.367)
  line L56 (-24.367, 64.367) -> (-23.7693, 66.5977)
  line L57 (-23.7693, 66.5977) -> (-25.4023, 68.2307)
  line L58 (-28.2307, 65.4023) -> (-25.6642, 62.8358)
  line L59 (-25.4023, 68.2307) -> (-22.8358, 65.6642)
  line L60 (0, 62.5) -> (-3.5, 66)
  line L61 (0, 66) -> (2.4749, 63.5251) construction
  line L62 (2.2307, 65.4023) -> (1.633, 67.633)
  line L63 (1.633, 67.633) -> (-0.5977, 68.2307)
  line L64 (-0.5977, 68.2307) -> (-2.2307, 66.5977)
  line L65 (-2.2307, 66.5977) -> (-1.633, 64.367)
  line L66 (-1.633, 64.367) -> (0.5977, 63.7693)
  line L67 (0.5977, 63.7693) -> (2.2307, 65.4023)
  line L68 (0.5977, 63.7693) -> (-0.3358, 62.8358)
  line L69 (-2.2307, 66.5977) -> (-3.1642, 65.6642)
  point P0 (-13, 33)
  point P1 (-13, 33)
  point P2 (-26, 0)
  point P3 (-26, 66)
  point P4 (0, 66)
  dimension "d224" = 2.5
  dimension "d225" = 26
  dimension "d226" = 66
  dimension "d227" = 2.5
  dimension "d228" = 2.5
  dimension "d229" = 2.5
  dimension "d234" = 7
  dimension "d235" = 7
  dimension "d236" = 7
  dimension "d237" = 7
  dimension "d238" = 30
  dimension "d239" = 70
  dimension "d240" = 2
  dimension "d241" = 45
  dimension "d242" = 2
  dimension "d243" = 45
  dimension "d244" = 45
  dimension "d245" = 2
  dimension "d246" = 45
  dimension "d247" = 2
  dimension "d248" = 2
  constraint coincident A0.centre L0.start
  constraint horizontal L0
  constraint vertical L1
  constraint horizontal L2
  constraint vertical L3
  constraint coincident P2 L0.end
  constraint coincident P3 L1.end
  constraint coincident P4 L2.end
  constraint concentric A0 A4
  constraint concentric A1 A5
  constraint concentric A2 A6
  constraint concentric A3 A7
  constraint horizontal L4
  constraint perpendicular L4 L5
  constraint parallel L4 L6
  constraint parallel L5 L7
  constraint coincident L8 P1
  constraint coincident L9 P1
  constraint horizontal L14
  constraint perpendicular L14 L15
  constraint parallel L14 L16
  constraint parallel L15 L17
  constraint coincident P1 P0
  constraint coincident L1 L18.start
  constraint coincident A5 L18.start
  constraint coincident L10 L18.end
  constraint tangent A5 L18
  constraint coincident A5 L19.start
  constraint coincident L0 L19.start
  constraint coincident L11 L19.end
  constraint tangent A5 L19
  constraint coincident A4 L20.start
  constraint coincident L0 L20.start
  constraint coincident L11 L20.end
  constraint tangent A4 L20
  constraint coincident A4 L21.start
  constraint coincident L3 L21.start
  constraint tangent A4 L21
  constraint coincident A6 L22.start
  constraint coincident L1 L22.start
  constraint coincident L10 L22.end
  constraint tangent A6 L22
  constraint coincident A6 L23.start
  constraint coincident L2 L23.start
  constraint coincident L13 L23.end
  constraint tangent A6 L23
  constraint coincident A7 L24.start
  constraint coincident L2 L24.start
  constraint coincident L13 L24.end
  constraint tangent A7 L24
  constraint coincident A7 L25.start
  constraint coincident L3 L25.start
  constraint coincident L12 L25.end
  constraint tangent A7 L25
  constraint horizontal L27
  constraint parallel L33 L34
  constraint horizontal L36
  constraint parallel L30 L35
  constraint coincident A5 L34.end
  constraint coincident A5 L35.end
  constraint horizontal L38
  constraint coincident A4 L37.end
  constraint coincident A4 L45.start
  constraint parallel L41 L45
  constraint coincident A4 L46.end
  constraint parallel L45 L46
  constraint perpendicular L47 L48
  constraint horizontal L51
  constraint coincident A6 L50.end
  constraint coincident L49 L58.end
  constraint perpendicular L49 L58
  constraint coincident L49 L59.end
  constraint perpendicular L49 L59
  constraint parallel L60 L61
  constraint coincident A7 L61.end
  constraint coincident L60 L68.end
  constraint perpendicular L60 L68
  constraint coincident L60 L69.end
  constraint perpendicular L60 L69
  measures "d224" diameter of A0
  measures "d225" distance of A0.centre L0.end
  measures "d226" distance of A0.centre P4
  measures "d227" diameter of A1
  measures "d228" diameter of A2
  measures "d229" diameter of A3
  measures "d234" diameter of A4
  measures "d235" diameter of A5
  measures "d236" diameter of A6
  measures "d237" diameter of A7
  measures "d238" distance of L5.end L6.end
  measures "d239" distance of L4.end L5.end
  measures "d241" angle of L26 L27
  measures "d242" distance of P2 L33
  measures "d243" angle of L35 L36
  measures "d244" angle of L37 L38
  measures "d245" distance of A0.centre L44
  measures "d246" angle of L50 L51
  measures "d247" distance of P3 L57
  measures "d248" distance of P4 L67
extrude "Rahmen" add sketch "Platine 3*7" against normal blind 3.6 separate body contours A0 L0 L3 L39 L40 L41 L42 L43 L44 L46 | A0 L0 L3 L39 L40 | L0 L3 L39 L40 L45 L46 L47 | L3 L39 L46 | L0 L40 L45 | L3 L46 L47 | L0 L3 A4 L41 L42 L43 L44 L45 L46 | L0 L45 L47 | A4 L11 L12 L20 L21 | L3 L60 L68 | L2 L3 A7 L62 L63 L64 L67 L68 L69 | A7 L12 L13 L24 L25 | L0 L1 A5 L30 L31 L32 L33 L34 L35 | A5 L10 L11 L18 L19 | L0 L34 L48 | L2 L3 L60 L65 L66 L68 L69 | L3 L66 L68 | L2 L60 L69 | L0 L28 L34 | L0 L1 L28 L29 L34 L35 L48 | L1 L35 L48 | L2 L3 A3 L65 L66 | L2 L3 A3 L62 L63 L64 L65 L66 L67 | L2 L49 L59 | L1 L2 A6 L52 L53 L54 L57 L58 L59 | A6 L10 L13 L22 L23 | L2 L65 L69 | L0 L1 A1 L28 L29 L30 L31 L32 L33 | L0 L1 A1 L28 L29 | L1 L49 L58 | L1 L29 L35 | L1 L2 L49 L55 L56 L58 L59 | L2 L56 L59 | L1 L55 L58 | L1 L2 A2 L55 L56 | L1 L2 A2 L52 L53 L54 L55 L56 L57 L58 L59 | L14 L15 L16 L17 makes body 11
extrude "Mutterhülsen" cut sketch "Platine 3*7" against normal blind 1.6 from surface at -1 contours A0 L0 L3 L39 L40 L41 L42 L43 L44 L46 | A0 L0 L3 L39 L40 | L0 L3 L39 L40 L45 L46 L47 | L3 L39 L46 | L0 L40 L45 | L2 L3 L60 L65 L66 L68 L69 | L3 L66 L68 | L0 L28 L34 | L0 L1 L28 L29 L34 L35 L48 | L2 L3 A3 L65 L66 | L2 L3 A3 L62 L63 L64 L65 L66 L67 | L2 L65 L69 | L0 L1 A1 L28 L29 L30 L31 L32 L33 | L0 L1 A1 L28 L29 | L1 L29 L35 | L1 L2 L49 L55 L56 L58 L59 | L2 L56 L59 | L1 L55 L58 | L1 L2 A2 L55 L56 | L1 L2 A2 L52 L53 L54 L55 L56 L57 L58 L59 bodies 11
hidden bodies 1 2 3 4 5 6 7 8 9 10
equation "d1 = ( 4 / 2 ) * 1 mm"
equation "d2 = ( 5,6 / 2 ) * 1 mm"
equation "d19 = ( 4,5 / 2 ) * 1 mm"
equation "d20 = ( 5,5 / 2 ) * 1 mm"
equation "d159 = 9,300 mm + 1,6 mm + 3 mm + 2 mm"
equation "d225 = 30 mm - 4 mm"
equation "d226 = 70 mm - 4 mm"
named bodies: "Einschubmutter M2", "Einschubmutter M3", "Eindrückmutter M2", "Eindrückmutter M3", "TOF", "USB-C Buchse", "USB-C Stecker", "ESP32-C6-DevKit-Case", "LED-Ring", "OLED SSD1306", "Platine 3*7"
